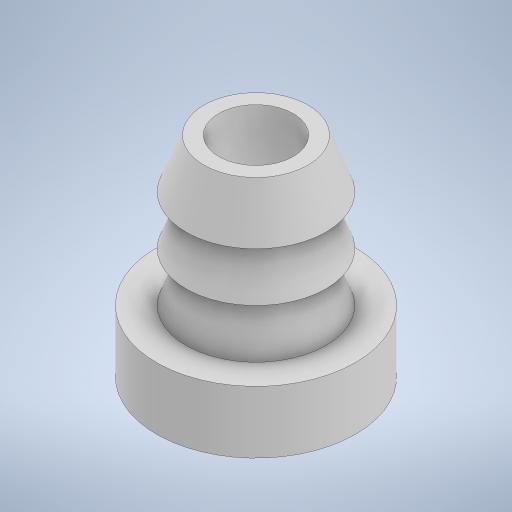
# Autodesk Inventor part: Hose Barb V4
Saved by Autodesk Inventor 2024.2 (Build 282272000, 272)
## iProperties
Created: 2024-08-10
Part Number: Hose Barb V4
Material: Generic
Document SubType Name: Modeling
Designer: balmo
Density: 1 g/cm^3
Appearance: Default
Author: balmo
## iProperties of the stored document Hose Barb_3DPrint.ipt
Created: 2024-08-10
Part Number: Hose Barb_3DPrint
Material: Generic
Document SubType Name: Modeling
Designer: balmo
Density: 1 g/cm^3
Appearance: Default
Author: balmo
Autodesk Inventor part; units mm, degrees
ref_plane "YZ Plane" through (0, 0, 0) normal (1, 0, 0) x (0, 1, 0)
ref_plane "XZ Plane" through (0, 0, 0) normal (0, 1, 0) x (-1, 0, 0)
ref_plane "XY Plane" through (0, 0, 0) normal (0, 0, 1) x (1, 0, 0)
sketch "Sketch1" plane through (0, 0, 0) normal (0, 0, 1) x (1, 0, 0)
  line L0 (0, 0) -> (3.5719, 0) construction
  line L1 (1.905, 7.5269) -> (1.905, 0)
  line L2 (1.905, 0) -> (3.5719, 0)
  line L3 (0, 0) -> (0, 5.4125) construction
  line L4 (3.5719, 0) -> (2.6587, 2.509)
  line L5 (2.6587, 2.509) -> (3.5719, 2.509)
  line L6 (3.5719, 2.509) -> (2.6587, 5.0179)
  line L7 (2.6587, 5.0179) -> (3.5719, 5.0179)
  line L8 (3.5719, 5.0179) -> (2.6587, 7.5269)
  line L9 (2.6587, 7.5269) -> (1.905, 7.5269)
  point P0 (2.0609, 0)
  dimension "d0" = 3.5719
  dimension "d4" = 1.905
  dimension "d9" = 70
  dimension "d12" = 70
  constraints: 20 end point, 4 horizontal, 2 point on line, 1 perpendicular, 1 vertical
  measures "d0" distance of L0.start L0.end
  measures "d4" distance between parallel lines of L1 L3
  measures "d9" angle of L4 L0
  measures "d12" angle of L8 L7
revolve "Revolution1" add sketch "Sketch1" angle 360 about axis through (0, 0, 0) along (0, 1, 0)
sketch "Sketch2" plane through (0, 0, 0) normal (0, -1, 0) x (1, 0, 0)
  circle A0 centre (0, 0) radius 5.08
  dimension "d5" = 10.16
  constraints: 1 centre point, 1 coincident
  measures "d5" diameter of A0
extrude "Extrusion1" add sketch "Sketch2" along normal blind 3.175
sketch "Sketch4" plane through (0, -3.175, 0) normal (0, -1, 0) x (1, 0, 0)
  circle A0 centre (0, 0) radius 1.905 projected
  circle A1 centre (0, -1.016) radius 0.762
  circle A2 centre (0.8799, 0.508) radius 0.762
  circle A3 centre (-0.8799, 0.508) radius 0.762
  dimension "d50" = 1.524
  dimension "d51" = 0.127
  dimension "d54" = 360
  constraints: 3 centre point, 7 other
  measures "d50" diameter of A1
extrude "Extrusion3" cut sketch "Sketch4" against normal through all contours A1 | A2 | A3
body "Solid1"
